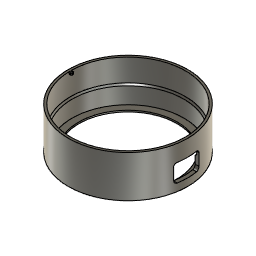
FlipwatchCase v2 (Autodesk Fusion 360 design; units mm, degrees)
Autodesk Fusion 360 part; units mm, degrees
note: some values were not read from the file. Set by a fixed rule: which sketch regions a step uses.
sketch "Esquisse4" plane through (0, 0, 0) normal (1, 0, 0) x (0, 1, 0)
  line L0 (40, 0) -> (40, 26)
  line L1 (33, 0) -> (33, 1)
  line L2 (33, 1) -> (37.5, 1)
  line L3 (37.5, 1) -> (37.5, 11)
  line L4 (38.5, 26) -> (40, 26)
  line L5 (33, 0) -> (40, 0)
  line L6 (37.5, 11) -> (37.5, 11.5)
  line L7 (38.5, 26) -> (38.5, 13)
  line L8 (37.5, 11.5) -> (37.5, 12.01)
  line L9 (38.49, 13) -> (38.5, 13)
  line L10 (37.5, 12.01) -> (38.49, 13)
  point P0 (37.5, 13)
  point P1 (37.5, 13)
  dimension "d14" = 1
  dimension "d16" = 7
  dimension "d17" = 40
  dimension "d18" = 10
  dimension "d20" = 26
  dimension "d22" = 2.5
  dimension "d26" = 1.5
  dimension "d27" = 0.99
  dimension "d28" = 0.99
  constraint vertical L0
  constraint perpendicular L1 L2
  constraint perpendicular L2 L3
  constraint coincident L0 L4.end
  constraint perpendicular L0 L4
  constraint perpendicular L0 L5
  constraint perpendicular L4 L7
  constraint coincident P1 L6
  constraint coincident P1 P0
  constraint perpendicular L7 L9
  constraint coincident P1 L8
  constraint coincident P1 L9
  measures "d14" distance of L1.start L1.end
  measures "d16" distance of L0.start L1.start
  measures "d17" distance of origin L0.start
  measures "d18" distance of L2.end L3.end
  measures "d20" distance of L0.start L0.end
  measures "d22" distance of L0 L3
  measures "d26" distance of L4.start L0.end
  measures "d27" distance of P1 L8.end
  measures "d28" distance of P1 L9.start
revolve "Révolution1" add sketch "Esquisse4" angle 360 about axis through (0, 0, 1.75) along (0, 0, 1)
sketch "Esquisse5" plane through (0, 0, 0) normal (1, 0, 0) x (0, 1, 0)
  line L0 (-6.5, 17) -> (6.5, 17)
  line L1 (8.5, 15) -> (8.5, 7)
  line L2 (6.5, 5) -> (-6.5, 5)
  line L3 (-8.5, 7) -> (-8.5, 15)
  line L4 (40, 0) -> (40, 26)
  line L5 (-40, 0) -> (40, 0)
  arc A0 (-6.5, 17) -> (-8.5, 15) centre (-6.5, 15) ccw
  arc A1 (8.5, 15) -> (6.5, 17) centre (6.5, 15) ccw
  arc A2 (6.5, 5) -> (8.5, 7) centre (6.5, 7) ccw
  arc A3 (-8.5, 7) -> (-6.5, 5) centre (-6.5, 7) ccw
  point P0 (-8.5, 17)
  point P1 (8.5, 17)
  point P2 (-8.5, 5)
  dimension "d29" = 17
  dimension "d30" = 12
  dimension "d31" = 31.5
  dimension "d33" = 5
  dimension "d34" = 2
  constraint horizontal L0
  constraint vertical L1
  constraint horizontal L2
  constraint vertical L3
  constraint coincident P0 L0
  constraint coincident P0 L3
  constraint tangent L0 A0
  constraint tangent L3 A0
  constraint coincident P1 L0
  constraint coincident P1 L1
  constraint tangent L0 A1
  constraint tangent L1 A1
  constraint equal A0 A1
  constraint tangent L1 A2
  constraint tangent L2 A2
  constraint equal A0 A2
  constraint coincident P2 L2
  constraint coincident P2 L3
  constraint tangent L2 A3
  constraint tangent L3 A3
  constraint equal A0 A3
  measures "d29" distance of P0 P1
  measures "d30" distance of P0 P2
  measures "d31" distance of L1 L4
  measures "d33" distance of L2 L5
  measures "d34" radius of A0
extrude "Extrusion4" cut sketch "Esquisse5" along normal blind 40
sketch "Esquisse6" plane through (0, 0, 26) normal (0, 0, 1) x (-1, 0, 0)
  circle A0 centre (0, 0) radius 38.5
  circle A1 centre (0, 0) radius 40
  circle A2 centre (0, 0) radius 40
  line L0 (38.487, -1) -> (36.987, -1)
  line L1 (78, 0) -> (-71.8724, 0) construction
  line L2 (36.987, -1) -> (36.987, 1)
  line L3 (36.987, 1) -> (38.487, 1)
  point P0 (38.487, -1)
  point P1 (38.487, 1)
  dimension "d38" = 80
  dimension "d39" = 1.5
  dimension "d40" = 1
  constraint horizontal L0
  constraint horizontal L1
  constraint perpendicular L1 L2
  constraint coincident A0 P1
  constraint perpendicular L2 L3
  constraint coincident P0 L0.start
  constraint coincident P1 L3.end
  measures "d38" diameter of A2
  measures "d39" distance of P0 L0.end
  measures "d40" distance of L0 L1
extrude "Extrusion5" add sketch "Esquisse6" along normal blind 2 contours A0 L0 L2 L3 | A1 A2 picked at (37.4913, 0)
fillet "Congé1" radius 0.6 8 edges at (-37.737, -1, 28) (-37.737, 1, 28) (-37.737, -1, 26) (-37.737, 1, 26) (-36.987, 1, 27) (-36.987, -1, 27) (-36.987, 0, 28) (-36.987, 0, 26)
equation "d28 = d27"
